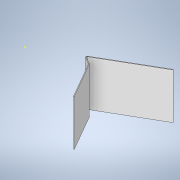
# Autodesk Inventor part: Soporte para libros
Saved by Autodesk Inventor 2022 (Build 260153000, 153)
## iProperties
Created: 2023-10-15
Part Number: Soporte para libros
Material: Generic
Document SubType Name: Sheet Metal
Designer: Administrador
Density: 1 g/cm^3
Sheet Metal Rule: Default
Appearance: Default
Flat Pattern Width: 20 cm
Flat Pattern Length: 50 cm
Flat Pattern Area: 1000 cm^2
Sheet Metal Width: 200.000 mm
Sheet Metal Length: 500.000 mm
Sheet Metal Area: 100000.000 mm^2
Author: Administrador
Autodesk Inventor part; units mm, degrees
ref_plane "YZ Plane" through (0, 0, 0) normal (1, 0, 0) x (0, 1, 0)
ref_plane "XZ Plane" through (0, 0, 0) normal (0, 1, 0) x (-1, 0, 0)
ref_plane "XY Plane" through (0, 0, 0) normal (0, 0, 1) x (1, 0, 0)
sketch "Sketch1" plane through (0, 0, 0) normal (0, 0, 1) x (1, 0, 0)
  line L0 (0, 0) -> (500, 0)
  line L1 (500, 0) -> (500, -200)
  line L2 (500, -200) -> (0, -200)
  line L3 (0, -200) -> (0, 0)
  dimension "d0" = 500
  dimension "d1" = 200
  measures "d0" distance of L1.end L2.end
  measures "d1" distance of L0.end L1.end
extrude "Plate1" add sketch "Sketch1" along normal blind 3.048
sketch "Sketch2" plane through (0, 0, 3.048) normal (0, 0, 1) x (1, 0, 0)
  line L0 (0, -200) -> (0, 0) projected
  line L1 (0, -200) -> (180, -200)
  line L2 (500, -200) -> (0, -200) projected
  line L3 (180, -200) -> (180, 0)
  line L4 (180, -200) -> (200, -200)
  line L5 (200, -200) -> (200, 0)
  line L6 (0, 0) -> (500, 0) projected
  dimension "d3" = 180
  dimension "d4" = 20
  constraints: 8 end point, 3 point on line, 2 perpendicular
  measures "d3" distance of L0.start L1.end
  measures "d4" distance of L1.end L4.end
fold "Fold1" angle 30 bend radius 3.048 thickness 3.048 k factor 0.44 line from (180, -200, 3.048) to (180, 0, 3.048) line at bend centre moving side (1, 0, 0) folds toward (0, 0, -1)
sketch "Sketch3" plane through (458.0319, -200, -157.1942) normal (0.5, 0, 0.8660254) x (0.8660254, 0, -0.5)
  line L0 (0, 0) -> (-318.8509, 0) projected
  line L1 (-318.8509, 0) -> (-278.8509, 0)
  line L2 (-278.8509, 0) -> (-278.8509, 200)
  line L3 (-318.8509, 200) -> (0, 200) projected
  point P0 (-475.2644, 200)
  dimension "d11" = 40
  constraints: 4 end point, 2 point on line, 1 perpendicular
  measures "d11" distance of L0.end L1.end
fold "Fold2" angle 120 bend radius 3.048 thickness 3.048 k factor 0.44 line from (216.5399, -200, -17.7687) to (216.5399, 0, -17.7687) line at bend centre moving side (-0.8660254, 0, 0.5) folds toward (0.5, 0, 0.8660254)
sketch "Sketch4" plane through (458.0319, -200, -157.1942) normal (0.5, 0, 0.8660254) x (0.8660254, 0, -0.5)
  point P0 (-475.2644, 200)
equation "\"d2\" = Thickness"
equation "\"d5\" = BendReliefWidth"
equation "\"d6\" = BendReliefDepth"
equation "\"d7\" = MinimumRemnant"
equation "\"d8\" = TransitionRadius"
equation "\"d10\" = BendRadius"
equation "\"d12\" = BendReliefWidth"
equation "\"d13\" = BendReliefDepth"
equation "\"d14\" = MinimumRemnant"
equation "\"d15\" = TransitionRadius"
equation "\"d17\" = BendRadius"
equation "\"BendRadius\" = Thickness"
equation "\"BendReliefWidth\" = Thickness"
equation "\"BendReliefDepth\" = 0.5 * Thickness"
equation "\"CornerReliefSize\" = 4 * Thickness"
equation "\"MinimumRemnant\" = 2 * Thickness"
equation "\"TransitionRadius\" = BendRadius"
equation "\"JacobiRadiusSize\" = BendRadius"
equation "\"GapSize\" = Thickness"
equation "\"Thickness\" = 3.048"
body "Solid1"
